Autodesk Fusion 360 part; units mm, degrees
(part 2 of 2)
  constraint coincident L87.end L88.start
  constraint coincident L83.end L84.start
  constraint horizontal L94
  constraint vertical L95
  constraint horizontal L96
  constraint vertical L97
  constraint horizontal L98
  constraint vertical L99
  constraint horizontal L100
  constraint vertical L101
  constraint horizontal L102
  constraint vertical L103
  constraint horizontal L104
  constraint vertical L105
  constraint horizontal L106
  constraint vertical L107
  constraint horizontal L108
  constraint vertical L109
  constraint horizontal L110
  constraint vertical L111
  constraint horizontal L112
  constraint vertical L113
  constraint horizontal L116
  constraint vertical L117
  constraint horizontal L114
  constraint vertical L115
  constraint horizontal L123
  constraint vertical L125
  constraint horizontal L124
  constraint vertical L122
  constraint horizontal L119
  constraint vertical L120
  constraint horizontal L121
  constraint vertical L118
  constraint vertical L131
  constraint vertical L129
  constraint horizontal L127
  constraint perpendicular L128 L129
  constraint perpendicular L126 L131
  constraint horizontal L130
  constraint vertical L134
  constraint vertical L141
  constraint horizontal L132
  constraint perpendicular L132 L133
  constraint parallel L132 L143
  constraint parallel L133 L142
  constraint tangent L132 A36
  constraint tangent A36 L133
  constraint tangent L132 A48
  constraint tangent L142 A48
  constraint tangent A35 L133
  constraint tangent A35 L143
  constraint tangent L142 A47
  constraint tangent L143 A47
  constraint vertical L140
  constraint vertical L137
  constraint horizontal L135
  constraint perpendicular L135 L139
  constraint parallel L135 L136
  constraint parallel L138 L139
  constraint tangent L135 A46
  constraint tangent A46 L139
  constraint tangent A39 L135
  constraint tangent A39 L138
  constraint tangent A45 L139
  constraint tangent L136 A45
  constraint tangent A40 L138
  constraint tangent A40 L136
  constraint horizontal L144
  constraint horizontal L145
  constraint horizontal L146
  constraint horizontal L147
  constraint vertical L151
  constraint vertical L149
  constraint horizontal L157
  constraint perpendicular L150 L157
  constraint parallel L155 L157
  constraint parallel L150 L156
  constraint tangent L157 A58
  constraint tangent L150 A58
  constraint tangent A51 L157
  constraint tangent A51 L156
  constraint tangent L150 A57
  constraint tangent L155 A57
  constraint tangent L156 A55
  constraint tangent L155 A55
  constraint vertical L158
  constraint vertical L152
  constraint horizontal L163
  constraint perpendicular L160 L163
  constraint parallel L153 L163
  constraint parallel L160 L162
  constraint tangent A62 L163
  constraint tangent L160 A62
  constraint tangent L163 A66
  constraint tangent L162 A66
  constraint tangent A59 L160
  constraint tangent L153 A59
  constraint tangent L162 A65
  constraint tangent L153 A65
  constraint horizontal L159
  constraint horizontal L148
  constraint horizontal L161
  constraint horizontal L154
  constraint vertical L164
  constraint vertical L168
  constraint horizontal L169
  constraint vertical L167
  constraint horizontal L165
  constraint horizontal L166
  constraint horizontal L170
  constraint vertical L171
  constraint horizontal L172
  constraint vertical L173
  constraint horizontal L174
  constraint vertical L175
  constraint horizontal L176
  constraint vertical L177
  constraint horizontal L178
  constraint vertical L179
  constraint horizontal L180
  constraint vertical L181
  constraint coincident L171.end L172.start
  constraint coincident L175.end L176.start
  constraint coincident L179.end L180.start
  constraint vertical L183
  constraint vertical L200
  constraint horizontal L196
  constraint perpendicular L190 L200
  constraint perpendicular L183 L202
  constraint horizontal L199
  constraint horizontal L189
  constraint vertical L182
  constraint horizontal L188
  constraint vertical L187
  constraint horizontal L201
  constraint vertical L203
  constraint horizontal L186
  constraint vertical L193
  constraint horizontal L198
  constraint vertical L195
  constraint horizontal L185
  constraint vertical L194
  constraint horizontal L192
  constraint vertical L197
  constraint horizontal L191
  constraint vertical L184
  constraint coincident A76.centre L191.start
  constraint coincident L182.end L188.start
  constraint coincident L186.start A78.centre
  constraint coincident L185.start L195.end
  constraint horizontal L204
  constraint vertical L205
  constraint horizontal L206
  constraint vertical L207
  constraint horizontal L208
  constraint vertical L209
  constraint horizontal L210
  constraint vertical L211
  constraint coincident P41 P13
  constraint coincident P14 P12
  constraint coincident P15 A85.centre
  constraint horizontal L213
  constraint vertical L212
  constraint horizontal L219
  constraint vertical L217
  constraint horizontal L215
  constraint vertical L214
  constraint horizontal L218
  constraint vertical L216
  constraint horizontal L220
  constraint vertical L221
  constraint horizontal L222
  constraint vertical L223
  constraint horizontal L224
  constraint perpendicular L224 L225
  constraint parallel L224 L226
  constraint parallel L225 L227
  constraint midpoint L213 P16
  constraint tangent L227 A87
  constraint tangent L224 A87
  constraint tangent L227 A88
  constraint tangent L226 A88
  constraint equal A87 A88
  constraint tangent L225 A89
  constraint tangent L226 A89
  constraint equal A87 A89
  constraint tangent L224 A90
  constraint tangent L225 A90
  constraint horizontal L228
  constraint vertical L229
  constraint horizontal L230
  constraint vertical L231
  constraint coincident P18 A95.centre
  constraint horizontal L238
  constraint vertical L239
  constraint horizontal L236
  constraint vertical L233
  constraint horizontal L234
  constraint perpendicular L234 L237
  constraint parallel L234 L235
  constraint parallel L232 L237
  constraint midpoint P17 L238
  constraint tangent A91 L232
  constraint tangent A91 L234
  constraint tangent L232 A92
  constraint tangent A92 L235
  constraint equal A91 A92
  constraint tangent A93 L237
  constraint tangent A93 L235
  constraint equal A91 A93
  constraint tangent L234 A96
  constraint tangent A96 L237
  constraint horizontal L240
  constraint vertical L241
  constraint horizontal L242
  constraint vertical L243
  constraint horizontal L244
  constraint vertical L245
  constraint horizontal L246
  constraint vertical L247
  constraint vertical L265
  constraint vertical L254
  constraint horizontal L269
  constraint vertical L263
  constraint horizontal L267
  constraint horizontal L260
  constraint coincident P21 A106.centre
  constraint horizontal L268
  constraint vertical L253
  constraint horizontal L266
  constraint vertical L249
  constraint horizontal L250
  constraint perpendicular L250 L258
  constraint parallel L250 L259
  constraint parallel L257 L258
  constraint midpoint P20 L268
  constraint tangent A105 L257
  constraint tangent A105 L250
  constraint tangent A104 L257
  constraint tangent A104 L259
  constraint equal A104 A105
  constraint tangent A108 L258
  constraint tangent A108 L259
  constraint equal A105 A108
  constraint tangent L250 A112
  constraint tangent A112 L258
  constraint horizontal L255
  constraint vertical L256
  constraint horizontal L248
  constraint vertical L252
  constraint horizontal L261
  constraint vertical L264
  constraint horizontal L262
  constraint vertical L251
  constraint coincident P24 A124.centre
  constraint horizontal L273
  constraint vertical L276
  constraint horizontal L282
  constraint vertical L287
  constraint horizontal L283
  constraint vertical L289
  constraint horizontal L286
  constraint vertical L285
  constraint horizontal L279
  constraint vertical L277
  constraint horizontal L270
  constraint vertical L278
  constraint horizontal L272
  constraint perpendicular L272 L274
  constraint parallel L271 L272
  constraint parallel L274 L280
  constraint midpoint P23 L273
  constraint tangent L280 A125
  constraint tangent L272 A125
  constraint tangent A119 L280
  constraint tangent L271 A119
  constraint equal A119 A125
  constraint tangent L274 A120
  constraint tangent L271 A120
  constraint equal A120 A125
  constraint tangent L272 A122
  constraint tangent L274 A122
  constraint horizontal L288
  constraint vertical L275
  constraint horizontal L281
  constraint vertical L284
  constraint coincident P44 P29
  constraint coincident P46 P30
  constraint coincident P33 P31
  constraint coincident P34 P32
  constraint horizontal L290
  constraint perpendicular L290 L291
  constraint parallel L290 L292
  constraint parallel L291 L293
  constraint coincident L294 P33
  constraint coincident L295 P33
  constraint horizontal L296
  constraint perpendicular L296 L297
  constraint parallel L296 L298
  constraint parallel L297 L299
  constraint coincident L300 P34
  constraint coincident L301 P34
  constraint horizontal L334
  constraint horizontal L331
  constraint tangent A133 L334
  constraint tangent A133 L331
  constraint tangent A134 L334
  constraint tangent A134 L331
  constraint horizontal L333
  constraint vertical L317
  constraint horizontal L332
  constraint vertical L319
  constraint horizontal L322
  constraint vertical L312
  constraint horizontal L307
  constraint vertical L318
  constraint horizontal L303
  constraint vertical L316
  constraint horizontal L302
  constraint vertical L304
  constraint horizontal L335
  constraint vertical L336
  constraint horizontal L323
  constraint vertical L326
  constraint horizontal L324
  constraint vertical L325
  constraint horizontal L309
  constraint vertical L310
  constraint horizontal L328
  constraint vertical L320
  constraint coincident L310.end A136.centre
  constraint coincident L303.start A131.centre
  constraint coincident A132.centre L324.start
  constraint coincident A130.centre L304.end
  constraint coincident P40 P37
  constraint coincident P39 P38
  constraint horizontal L327
  constraint perpendicular L308 L327
  constraint parallel L321 L327
  constraint parallel L308 L311
  constraint coincident P40 L330
  constraint coincident P40 L329
  constraint horizontal L315
  constraint perpendicular L306 L315
  constraint parallel L315 L337
  constraint parallel L306 L313
  constraint coincident P39 L314
  constraint coincident P39 L305
  constraint horizontal L348
  constraint vertical L346
  constraint horizontal L349
  constraint vertical L350
  constraint horizontal L347
  constraint horizontal L339
  constraint vertical L338
  constraint horizontal L340
  constraint vertical L342
  constraint horizontal L344
  constraint vertical L343
  constraint horizontal L345
  constraint vertical L341
  constraint horizontal L354
  constraint vertical L351
  constraint horizontal L352
  constraint vertical L353
  constraint horizontal L355
  constraint vertical L357
  constraint horizontal L356
  constraint vertical L358
  constraint coincident A140.centre L356.start
  constraint coincident L338.end L340.start
  constraint coincident L351.end L352.start
  constraint coincident A137.centre L343.end
  constraint horizontal L359
  constraint perpendicular L359 L360
  constraint parallel L359 L361
  constraint parallel L360 L362
  constraint coincident L363 P41
  constraint coincident L364 P41
  constraint horizontal L365
  constraint perpendicular L365 L366
  constraint parallel L365 L367
  constraint parallel L366 L368
  constraint coincident L369 P43
  constraint coincident L370 P43
  constraint coincident P43 P42
  constraint midpoint L42 L371.start
  constraint midpoint L40 L371.end
  constraint symmetric L359.start L371 L372.start
  constraint symmetric L359.end L371 L372.end
  constraint symmetric L360.end L371 L373.end
  constraint symmetric L361.end L371 L374.start
  constraint symmetric L365.start L371 L378.start
  constraint symmetric L365.end L371 L376.start
  constraint symmetric L366.end L371 L376.end
  constraint symmetric L367.end L371 L377.end
  constraint horizontal L380
  constraint perpendicular L380 L381
  constraint parallel L380 L382
  constraint parallel L381 L383
  constraint coincident L384 P44
  constraint coincident L385 P44
  constraint horizontal L386
  constraint perpendicular L386 L387
  constraint parallel L386 L388
  constraint parallel L387 L389
  constraint coincident L390 P45
  constraint coincident L391 P45
  constraint horizontal L392
  constraint perpendicular L392 L393
  constraint parallel L392 L394
  constraint parallel L393 L395
  constraint coincident L396 P46
  constraint coincident L397 P46
  constraint symmetric L35 L38.end L402.end
  constraint symmetric L35 L38.start L402.start
  constraint symmetric L35 L39.start L412.start
  constraint symmetric L35 L39.end L412.end
  constraint symmetric L35 P46 P51
  constraint symmetric L35 P44 P53
  constraint symmetric L35 L380.start L400.start
  constraint symmetric L35 L380.end L400.end
  constraint symmetric L35 L381.end L404.end
  constraint symmetric L35 L382.end L409.end
  constraint symmetric L35 L386.start L399.start
  constraint symmetric L35 L386.end L401.start
  constraint symmetric L35 L387.end L398.start
  constraint symmetric L35 L388.end L398.end
  constraint symmetric L35 P45 P52
  constraint symmetric L35 L392.start L405.end
  constraint symmetric L35 L392.end L406.end
  constraint symmetric L35 L393.end L410.start
  constraint symmetric L35 L394.end L405.start
  constraint coincident P60 P59
  constraint coincident P61 P58
  constraint horizontal L430
  constraint perpendicular L420 L430
  constraint parallel L421 L430
  constraint parallel L420 L425
  constraint coincident P60 L422
  constraint coincident P60 L426
  constraint horizontal L428
  constraint perpendicular L419 L428
  constraint parallel L423 L428
  constraint parallel L419 L431
  constraint coincident P55 L429
  constraint coincident P55 L427
  constraint horizontal L433
  constraint perpendicular L432 L433
  constraint parallel L433 L434
  constraint parallel L432 L435
  constraint coincident P61 L436
  constraint coincident P61 L418
  constraint coincident P54 L420.end
  constraint midpoint L332 L438.end
  constraint perpendicular L332 L438
  constraint symmetric P54 L438 P66
  constraint symmetric L424.start L438 L456.start
  constraint symmetric L424.end L438 L456.end
  constraint symmetric L437.start L438 L444.start
  constraint symmetric L437.end L438 L444.end
  constraint symmetric L419.start L438 L450.start
  constraint symmetric L418.end L438 L442.start
  constraint symmetric L418.start L438 L443.end
  constraint symmetric L428.start L438 L445.end
  constraint symmetric L433.start L438 L442.end
  constraint symmetric L423.end L438 L445.start
  constraint symmetric P55 L438 P62
  constraint symmetric P60 L438 P67
  constraint symmetric L419.end L438 L450.end
  constraint symmetric L422.start L438 L439.start
  constraint symmetric L421.end L438 L440.start
  constraint symmetric P61 L438 P69
  constraint symmetric L420.start L438 L439.end
  constraint symmetric L432.end L438 L447.end
  constraint coincident A53.centre L459.end
  constraint coincident L159 L460.end
  constraint perpendicular L159 L460
  measures "d11" radius of A0
  measures "d12" distance of L4.end L5.end
  measures "d13" distance of L6.end L7.end
  measures "d14" distance of L5.end L4.end
  measures "d15" distance of L6.end L7.end
  measures "d16" distance of L0.end L15.end
  measures "d17" distance of L0.start L16.end
  measures "d19" distance of L1.end L19.end
  measures "d22" diameter of A3
  measures "d23" diameter of A4
  measures "d24" diameter of A5
  measures "d25" diameter of A6
  measures "d26" diameter of A7
  measures "d27" distance of L22.start L23.end
  measures "d28" distance of L23.end L24.end
  measures "d29" distance of L24.end L25.end
  measures "d33" diameter of A8
  measures "d34" diameter of A9
  measures "d35" diameter of A10
  measures "d36" diameter of A11
  measures "d37" diameter of A12
  measures "d38" diameter of A13
  measures "d39" diameter of A14
  measures "d43" distance of L30.start L32.end
  measures "d63" distance of L30.start L36.start
  measures "d64" distance of A0.centre A1.centre
  measures "d65" distance of L35.end A0.centre
  measures "d83" distance of L38.end L38.start
  measures "d84" distance of L39.start L39.end
  measures "d85" distance of L38.start L39.end
  measures "d194" distance of L40.start L42.end
  measures "d195" distance of L45.start L44.end
  measures "d196" distance of L44.start L44.end
  measures "d350" distance of L49.end L49.start
  measures "d352" distance of L57.start L54.end
  measures "d357" distance of L48.end L59.end
  measures "d358" distance of L48.start L60.end
  measures "d359" distance of L49.end L61.end
  measures "d360" distance of L49.start L62.end
  measures "d361" distance of L68.start L64.start
  measures "d362" distance of L68.start L70.end
  measures "d363" distance of L67.start L71.end
  measures "d364" distance of L63.start L63.end
  measures "d365" distance of L64.start L64.end
  measures "d366" distance of L68.start L76.end
  measures "d367" distance of L70.end L73.end
  measures "d368" radius of A15
  measures "d369" radius of A16
  measures "d370" radius of A17
  measures "d371" radius of A18
  measures "d372" radius of A19
  measures "d373" radius of A20
  measures "d374" radius of A21
  measures "d375" radius of A22
  measures "d376" diameter of A23
  measures "d377" diameter of A24
  measures "d378" diameter of A25
  measures "d379" diameter of A26
  measures "d380" diameter of A27
  measures "d381" diameter of A28
  measures "d382" diameter of A29
  measures "d383" diameter of A30
  measures "d384" distance of L30.end L78.end
  measures "d385" distance of L30.end L80.end
  measures "d387" distance of L31.end L84.end
  measures "d389" distance of L32.end L88.end
  measures "d390" distance of L30.start L90.end
  measures "d391" distance of L30.start L92.end
  measures "d392" diameter of A31
  measures "d393" diameter of A32
  measures "d394" diameter of A33
  measures "d395" diameter of A34
  measures "d537" distance of L30.start L30.end
  measures "d553" distance of L94.start L96.end
  measures "d554" distance of L98.start L100.end
  measures "d555" distance of L102.start L104.end
  measures "d556" distance of L106.start L108.end
  measures "d807" distance of L128.end L129.start
  measures "d858" radius of A36
  measures "d859" radius of A48
  measures "d860" radius of A35
  measures "d861" radius of A47
  measures "d862" diameter of A38
  measures "d863" diameter of A49
  measures "d865" diameter of A37
  measures "d876" radius of A46
  measures "d877" radius of A39
  measures "d878" radius of A45
  measures "d879" radius of A40
  measures "d880" diameter of A44
  measures "d881" diameter of A42
  measures "d882" diameter of A41
  measures "d883" diameter of A43
  measures "d884" diameter of A50
  measures "d892" radius of A58
  measures "d893" radius of A51
  measures "d894" radius of A57
  measures "d895" radius of A55
  measures "d896" diameter of A53
  measures "d897" diameter of A54
  measures "d898" diameter of A56
  measures "d899" radius of A62
  measures "d900" radius of A66
  measures "d901" radius of A59
  measures "d902" radius of A65
  measures "d903" diameter of A64
  measures "d904" diameter of A60
  measures "d905" diameter of A63
  measures "d906" diameter of A61
  measures "d907" diameter of A52
  measures "d934" distance of L137.end L137.start
  measures "d943" diameter of A67
  measures "d944" diameter of A68
  measures "d945" distance of L126.end L170.end
  measures "d946" distance of L126.end L172.end
  measures "d947" distance of L128.end L174.end
  measures "d948" distance of L128.end L176.end
  measures "d949" distance of L129.start L178.end
  measures "d950" distance of L129.start L180.end
  measures "d954" diameter of A73
  measures "d955" diameter of A74
  measures "d956" diameter of A75
  measures "d957" distance of L194.end L190.end
  measures "d959" distance of L187.start L183.end
  measures "d961" distance of L186.end L190.end
  measures "d962" distance of L195.start L194.end
  measures "d963" distance of L185.end L194.end
  measures "d964" distance of L192.end L183.start
  measures "d965" distance of L184.start L183.start
  measures "d966" diameter of A76
  measures "d967" diameter of A77
  measures "d968" diameter of A78
  measures "d969" diameter of A79
  measures "d981" distance of L40.start L206.end
  measures "d983" distance of L40.end L210.end
  measures "d1011" diameter of A80
  measures "d1012" diameter of A86
  measures "d1013" diameter of A83
  measures "d1014" diameter of A81
  measures "d1015" diameter of A85
  measures "d1016" diameter of A84
  measures "d1017" diameter of A82
  measures "d1018" distance of L213.start L215.start
  measures "d1019" distance of L215.start L214.start
  measures "d1020" distance of L215.start L216.start
  measures "d1049" distance of L213.start L212.start
  measures "d1050" distance of L212.end L212.start
  measures "d1051" distance of L212.start L220.end
  measures "d1052" distance of L212.start L222.end
  measures "d1055" radius of A87
  measures "d1056" radius of A90
  measures "d1057" distance of L228.start L221.end
  measures "d1058" distance of L228.start L214.end
  measures "d1059" diameter of A97
  measures "d1060" diameter of A94
  measures "d1061" diameter of A101
  measures "d1062" diameter of A100
  measures "d1063" diameter of A95
  measures "d1064" diameter of A98
  measures "d1065" diameter of A99
  measures "d1066" distance of L233.start L233.end
  measures "d1069" distance of L238.end L233.end
  measures "d1072" radius of A91
  measures "d1073" radius of A96
  measures "d1074" distance of L238.end L240.end
  measures "d1075" distance of L238.end L242.end
  measures "d1076" distance of L233.start L244.end
  measures "d1077" distance of L233.start L246.end
  measures "d1094" diameter of A116
  measures "d1095" diameter of A118
  measures "d1096" diameter of A111
  measures "d1097" diameter of A113
  measures "d1098" diameter of A103
  measures "d1099" diameter of A107
  measures "d1100" diameter of A106
  measures "d1101" diameter of A109
  measures "d1102" diameter of A102
  measures "d1103" distance of L249.start L249.end
  measures "d1104" distance of L252.end L249.end
  measures "d1105" radius of A105
  measures "d1106" radius of A112
  measures "d1107" distance of L255.end L252.end
  measures "d1108" distance of L252.end L248.end
  measures "d1109" distance of L261.end L249.start
  measures "d1110" distance of L251.start L249.start
  measures "d1111" diameter of A126
  measures "d1112" diameter of A129
  measures "d1113" diameter of A121
  measures "d1114" diameter of A123
  measures "d1115" diameter of A124
  measures "d1116" diameter of A128
  measures "d1117" diameter of A127
  measures "d1118" distance of L282.end L273.start
  measures "d1119" distance of L282.end L283.end
  measures "d1120" distance of L282.end L285.start
  measures "d1121" distance of L273.end L273.start
  measures "d1122" distance of L273.end L277.start
  measures "d1123" distance of L270.end L273.end
  measures "d1124" radius of A125
  measures "d1125" radius of A122
  measures "d1126" distance of L284.end L270.start
  measures "d1127" distance of L284.end L281.end
  measures "d1144" distance of L291.end L292.end
  measures "d1145" distance of L290.end L291.end
  measures "d1146" distance of L297.end L298.end
  measures "d1147" distance of L296.end L297.end
  measures "d1148" radius of A133
  measures "d1171" distance of L319.start L309.start
  measures "d1174" distance of L309.start L312.start
  measures "d1187" distance of L307.start L307.end
  measures "d1188" distance of L307.start L303.end
  measures "d1189" distance of L302.start L335.end
  measures "d1190" distance of L319.start L324.end
  measures "d1191" distance of L309.start L309.end
  measures "d1192" distance of L309.start L320.start
  measures "d1193" diameter of A136
  measures "d1194" diameter of A131
  measures "d1195" diameter of A132
  measures "d1196" diameter of A130
  measures "d1197" distance of L307.start L309.start
  measures "d1210" distance of L308.end L311.start
  measures "d1211" distance of L308.end L308.start
  measures "d1212" distance of L305.end L306.end
  measures "d1213" distance of L305.start L306.end
  measures "d1237" distance of L349.end L347.start
  measures "d1253" distance of L339.start L338.start
  measures "d1254" distance of L339.start L340.end
  measures "d1255" distance of L341.end L341.start
  measures "d1256" distance of L349.end L352.end
  measures "d1257" distance of L347.start L355.end
  measures "d1258" distance of L347.start L356.end
  measures "d1259" diameter of A140
  measures "d1260" diameter of A138
  measures "d1261" diameter of A139
  measures "d1262" diameter of A137
  measures "d1263" distance of L339.start L347.start
  measures "d1322" distance of L360.end L361.end
  measures "d1323" distance of L359.end L360.end
  measures "d1324" distance of L366.end L367.end
  measures "d1325" distance of L365.end L366.end
  measures "d1326" distance of L381.end L382.end
  measures "d1327" distance of L380.end L381.end
  measures "d1328" distance of L387.end L388.end
  measures "d1329" distance of L386.end L387.end
  measures "d1330" distance of L393.end L394.end
  measures "d1331" distance of L392.end L393.end
  measures "d1332" distance of L424.start L424.end
  measures "d1333" distance of L437.start L437.end
  measures "d1334" distance of L424.start L437.end
  measures "d1335" distance of P54 L421.end
  measures "d1336" distance of P54 L420.start
  measures "d1337" distance of L423.end L419.end
  measures "d1338" distance of L419.start L419.end
  measures "d1339" distance of L418.end L432.end
  measures "d1340" distance of L418.start L432.end
  measures "d1347" diameter of A141
extrude "돌출62" add sketch "스케치1" along normal blind 5 contours L317 L319 L332 L333 makes body 1
extrude "돌출63" add sketch "스케치1" along normal blind 9 separate body contours L30 L31 L32 L33 | L40 L41 L42 L43 | L44 L45 L46 L47 | L66 L68 L70 L75 | L94 L95 L96 L97 | L98 L99 L100 L101 | L102 L103 L104 L105 | L106 L107 L108 L109 | L110 L111 L112 L113 | L114 L115 L116 L117 | L118 L119 L120 L121 | L122 L123 L124 L125 | L126 L127 L128 L129 L130 L131 | L134 L141 L144 L145 | L148 L149 L151 A53 L159 L459 L460 | A53 L159 L459 L460 | L164 L165 L166 L167 L168 | L183 L190 L196 L199 L200 L202 | L228 L229 L230 L231 | L254 L260 L263 L265 L267 | L275 L281 L284 L288 | L346 L348 L349 L350 | A141 makes body 2 at (1528.4276, -1089.433, 0) makes body 3 at (813.4968, -867.598, 0) makes body 4 at (1340.4245, -1498.5046, 0) makes body 5 at (624.4965, -1590.7079, 0) makes body 6 at (435.1019, 338.1172, 0) makes body 7 at (241.3333, -481, 0) makes body 8 at (264.4965, -1590.7079, 0) makes body 9 at (1170.9143, -1087.2127, 0) makes body 10 at (1163.4968, -867.598, 0) makes body 11 at (1550.7609, -1439.433, 0) makes body 12 at (1751.5009, -955.9592, 0) makes body 13 at (1428.4276, -1089.433, 0) makes body 14 at (813.4968, -1667.598, 0) makes body 15 at (990.4245, -1498.5046, 0) makes body 16 at (50.5, -1292, 0) makes body 17 at (348.4329, -826.6931, 0) makes body 18 at (221.3333, -1446.3333, 0) makes body 19 at (813.2197, -1078.1319, 0) makes body 20 at (1163.4968, -1667.598, 0) makes body 21 at (1450.7609, -1439.433, 0) makes body 22 at (1811.5009, -1585.9592, 0)
move_body "정렬110" bodies 7 to x (1, 0, 0) y (0, 1, 0) z (0, 0, 1) at (0, 725, 9)
move_body "이동82" bodies 16 8 5 18 to x (1, 0, 0) y (0, 0, 1) z (0, -1, 0) at (0, -1213.5, 1218.5)
move_body "이동83" bodies 5 8 to x (0, -1, 0) y (1, 0, 0) z (0, 0, 1) at (1446.3298, -980.6702, 0)
move_body "정렬111" bodies 5 to x (1, 0, 0) y (0, 1, 0) z (0, 0, 1) at (431.1702, 1862, 426.7079)
move_body "정렬112" bodies 8 to x (1, 0, 0) y (0, 1, 0) z (0, 0, 1) at (-223.8298, 1502, 426.7079)
move_body "정렬113" bodies 16 to x (1, 0, 0) y (0, 1, 0) z (0, 0, 1) at (0, 1738.5, 132.5)
move_body "정렬114" bodies 18 to x (1, 0, 0) y (0, 1, 0) z (0, 0, 1) at (0, 1456.5, 294.5)
move_body "정렬115" bodies 17 to x (1, 0, 0) y (0, 1, 0) z (0, 0, 1) at (0, 1100, 91)
move_body "정렬116" bodies 1 to x (1, 0, 0) y (0, 1, 0) z (0, 0, 1) at (0, 1450, 100)
move_body "이동84" bodies 3 10 12 20 22 9 4 19 15 14 to x (0, -1, 0) y (1, 0, 0) z (0, 0, 1) at (1628.7615, -195.7679, 0)
move_body "이동85" bodies 12 15 19 4 9 22 to x (0, 0, 1) y (0, 1, 0) z (-1, 0, 0) at (630.3286, 0, -630.3286)
move_body "정렬117" bodies 22 to x (1, 0, 0) y (0, 1, 0) z (0, 0, 1) at (-9, 569.5041, 317.5262)
move_body "정렬118" bodies 10 to x (1, 0, 0) y (0, 1, 0) z (0, 0, 1) at (-171.1683, 0, -280)
move_body "정렬119" bodies 4 to x (1, 0, 0) y (0, 1, 0) z (0, 0, 1) at (-85, 0, 339)
move_body "정렬120" bodies 15 to x (1, 0, 0) y (0, 1, 0) z (0, 0, 1) at (42.6714, 1437.2647, 619)
move_body "정렬121" bodies 14 to x (1, 0, 0) y (0, 1, 0) z (0, 0, 1) at (756.5032, 1437.2647, 0)
move_body "정렬122" bodies 12 to x (1, 0, 0) y (0, 1, 0) z (0, 0, 1) at (118.6714, 2356.7688, 247.5262)
move_body "정렬123" bodies 19 to x (1, 0, 0) y (0, 1, 0) z (0, 0, 1) at (127.6714, 1437.2647, 280)
move_body "정렬124" bodies 20 to x (1, 0, 0) y (0, 1, 0) z (0, 0, 1) at (756.5032, 1787.2647, 291)
move_body "정렬125" bodies 4 to x (1, 0, 0) y (0, 1, 0) z (0, 0, 1) at (-545.3286, 1787.2647, 280)
move_body "정렬126" bodies 10 to x (1, 0, 0) y (0, 1, 0) z (0, 0, 1) at (-621.3286, 1787.2647, 280)
move_body "정렬127" bodies 22 to x (1, 0, 0) y (0, 1, 0) z (0, 0, 1) at (-697.3286, 1787.2647, 280)
move_body "정렬128" bodies 9 to x (1, 0, 0) y (0, 1, 0) z (0, 0, 1) at (-715.3286, 1787.2647, 280)
move_body "정렬129" bodies 3 to x (1, 0, 0) y (0, 1, 0) z (0, 0, 1) at (-792.4968, 1437.2647, 291)
move_body "이동86" bodies 11 13 21 2 to x (1, 0, 0) y (0, 0, 1) z (0, -1, 0) at (0, -1481.933, 1490.933)
move_body "정렬130" bodies 21 to x (1, 0, 0) y (0, 1, 0) z (0, 0, 1) at (-733.0943, 1724.933, 145.5)
move_body "정렬131" bodies 11 to x (1, 0, 0) y (0, 1, 0) z (0, 0, 1) at (-833.0943, 2006.933, 145.5)
move_body "정렬132" bodies 2 to x (1, 0, 0) y (0, 1, 0) z (0, 0, 1) at (-1582.0943, 2006.933, -204.5)
move_body "정렬133" bodies 13 to x (1, 0, 0) y (0, 1, 0) z (0, 0, 1) at (-1482.0943, 1724.933, -204.5)
equation "d1077 = 26.5 mm - 9 mm"
